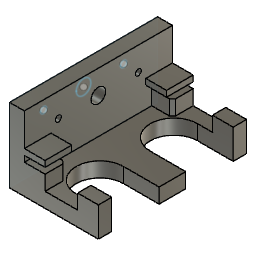
Ultrasonic sensor mount v1 (Autodesk Fusion 360 design; units mm, degrees)
Autodesk Fusion 360 part; units mm, degrees
sketch "Sketch1" plane through (0, 0, 0) normal (0, 0, 1) x (1, 0, 0)
  line L0 (0, 0) -> (30, 0)
  line L1 (30, 0) -> (30, 50)
  line L2 (30, 50) -> (0, 50)
  line L3 (0, 50) -> (0, 0)
  dimension "d1" = 30
  dimension "d2" = 50
  constraint horizontal L0
  constraint vertical L1
  constraint horizontal L2
  constraint vertical L3
  constraint coincident L0.start L3.end
  measures "d1" distance of L0.start L0.end
  measures "d2" distance of L0.start L2.end
extrude "Extrude1" add sketch "Sketch1" along normal blind 5
sketch "Sketch2" plane through (0, 0, 5) normal (0, 0, 1) x (-1, 0, 0)
  line L0 (0, -50) -> (0, 0)
  line L1 (0, 0) -> (-30, 0)
  line L2 (-30, 0) -> (-30, -50)
  line L3 (-30, -50) -> (0, -50)
  line L4 (0, -50) -> (-5, -50)
  line L5 (-5, -50) -> (-5, 0)
  line L6 (-5, 0) -> (0, 0)
  line L7 (0, 0) -> (0, -50)
  constraint horizontal L4
  constraint vertical L5
  constraint horizontal L6
  constraint vertical L7
  constraint coincident L0.start L3.end
extrude "Extrude2" add sketch "Sketch2" along normal blind 20 contours L0 L1 L3 L4 L5 L6 L7
sketch "Sketch3" plane through (0, 0, 5) normal (0, 0, 1) x (-1, 0, 0)
  line L0 (-5, -50) -> (-5, 0)
  line L1 (-5, 0) -> (-30, 0)
  line L2 (-30, 0) -> (-30, -50)
  line L3 (-30, -50) -> (-5, -50)
  line L4 (-30, 0) -> (-23, 0)
  line L5 (-23, 0) -> (-23, -7)
  line L6 (-23, -7) -> (-30, -7)
  line L7 (-30, -7) -> (-30, 0)
  line L8 (-30, -50) -> (-23, -50)
  line L9 (-23, -50) -> (-23, -43)
  line L10 (-23, -43) -> (-30, -43)
  line L11 (-30, -43) -> (-30, -50)
  line L12 (-5, -50) -> (-12, -50)
  line L13 (-12, -50) -> (-12, -43)
  line L14 (-12, -43) -> (-5, -43)
  line L15 (-5, -43) -> (-5, -50)
  line L16 (-5, 0) -> (-12, 0)
  line L17 (-12, 0) -> (-12, -7)
  line L18 (-12, -7) -> (-5, -7)
  line L19 (-5, -7) -> (-5, 0)
  circle A0 centre (-18, -12.5) radius 8
  circle A1 centre (-18, -37.5) radius 8
  dimension "d7" = 7
  dimension "d8" = 7
  dimension "d9" = 7
  dimension "d10" = 7
  dimension "d11" = 7
  dimension "d12" = 7
  dimension "d13" = 7
  dimension "d14" = 7
  dimension "d16" = 16
  dimension "d17" = 16
  constraint horizontal L4
  constraint vertical L5
  constraint horizontal L6
  constraint vertical L7
  constraint coincident L1.end L2.start
  constraint horizontal L8
  constraint vertical L9
  constraint horizontal L10
  constraint vertical L11
  constraint coincident L2.end L3.start
  constraint horizontal L12
  constraint vertical L13
  constraint horizontal L14
  constraint vertical L15
  constraint coincident L0.start L3.end
  constraint horizontal L16
  constraint vertical L17
  constraint horizontal L18
  constraint vertical L19
  constraint coincident L0.end L1.start
  measures "d7" distance of L1.end L4.end
  measures "d8" distance of L1.end L6.end
  measures "d9" distance of L2.end L8.end
  measures "d10" distance of L2.end L10.end
  measures "d11" distance of L0.start L12.end
  measures "d12" distance of L0.start L14.end
  measures "d13" distance of L0.end L16.end
  measures "d14" distance of L0.end L18.end
  measures "d16" diameter of A0
  measures "d17" diameter of A1
extrude "Extrude3" cut sketch "Sketch3" against normal blind 5 contours L9 L10 A1 | L5 L6 A0 picked at (-16.0576, -35.427) picked at (-16.0576, -14.573)
extrude "Extrude4" add sketch "Sketch3" along normal blind 5 contours L0 L3 L12 L13 L14 L15 | L0 L1 L16 L17 L18 L19 | L2 L3 L8 L9 L10 L11 A1 | L1 L2 L4 L5 L6 L7 A0
extrude "Extrude5" cut sketch "Sketch3" against normal blind 5 contours L9 L10 A1 | L5 L6 A0 picked at (-23.2774, -43.2566) picked at (-23.2774, -6.7434)
chamfer "Chamfer1" distance 1 angle 45 2 edges at (12, 7, 7.5) (12, 43, 7.5)
sketch "Sketch4" plane through (30, 0, 0) normal (1, 0, 0) x (0, 1, 0)
  line L0 (0, 0) -> (50, 0)
  line L1 (50, 0) -> (50, 10)
  line L2 (50, 10) -> (43, 10)
  line L3 (43, 10) -> (43, 5)
  line L4 (43, 5) -> (7, 5)
  line L5 (7, 5) -> (7, 10)
  line L6 (7, 10) -> (0, 10)
  line L7 (0, 10) -> (0, 0)
  line L8 (20.5, 5.0863) -> (4.5107, 5.0863)
  line L9 (4.5107, 5.0863) -> (4.5107, 0)
  line L10 (4.5107, 0) -> (20.5, 0)
  line L11 (20.5, 0) -> (20.5, 5.0863)
  line L12 (29.4867, 0) -> (45.5, 0)
  line L13 (45.5, 0) -> (45.5, 5.0968)
  line L14 (45.5, 5.0968) -> (29.4867, 5.0968)
  line L15 (29.4867, 5.0968) -> (29.4867, 0)
  line L16 (7, 10) -> (4.5107, 10)
  line L17 (4.5107, 10) -> (4.5107, 5.0863)
  line L18 (4.5107, 5.0863) -> (7, 5.0863)
  line L19 (7, 5.0863) -> (7, 10)
  line L20 (43, 10) -> (45.5, 10)
  line L21 (45.5, 10) -> (45.5, 5.0968)
  line L22 (45.5, 5.0968) -> (43, 5.0968)
  line L23 (43, 5.0968) -> (43, 10)
  constraint horizontal L8
  constraint vertical L9
  constraint horizontal L10
  constraint vertical L11
  constraint coincident L0 L9.end
  constraint horizontal L12
  constraint vertical L13
  constraint horizontal L14
  constraint vertical L15
  constraint coincident L0 L12.start
  constraint horizontal L16
  constraint vertical L17
  constraint horizontal L18
  constraint vertical L19
  constraint coincident L5.end L6.start
  constraint horizontal L20
  constraint vertical L21
  constraint horizontal L22
  constraint vertical L23
  constraint coincident L2.end L3.start
extrude "Extrude6" cut sketch "Sketch4" against normal blind 12 contours L0 L4 L5 L8 L9 L10 L11 L18 | L5 L6 L8 L16 L17 L18 L19 | L0 L3 L4 L12 L13 L14 L15 L22 | L2 L3 L14 L20 L21 L22 L23
sketch "Sketch5" plane through (0, 0, 0) normal (-1, 0, 0) x (0, -1, 0)
  line L0 (-50, 0) -> (0, 0)
  line L1 (0, 0) -> (0, 25)
  line L2 (0, 25) -> (-50, 25)
  line L3 (-50, 25) -> (-50, 0)
  circle A0 centre (-25, 17) radius 2.45
  circle A1 centre (-38.5, 17) radius 1
  circle A2 centre (-11.5, 17) radius 1
  dimension "d27" = 4.9
  dimension "d36" = 2
  dimension "d37" = 2
  measures "d27" diameter of A0
  measures "d36" diameter of A1
  measures "d37" diameter of A2
extrude "Extrude7" cut sketch "Sketch5" against normal blind 5 contours A0 | A1 | A2
sketch "Sketch6" plane through (5, 0, 0) normal (1, 0, 0) x (0, 1, 0)
  circle A0 centre (25, 17) radius 2.45
  line L0 (0, 10) -> (7, 10)
  line L1 (7, 10) -> (7, 5)
  line L2 (7, 5) -> (43, 5)
  line L3 (43, 5) -> (43, 10)
  line L4 (43, 10) -> (50, 10)
  line L5 (50, 10) -> (50, 25)
  line L6 (50, 25) -> (0, 25)
  line L7 (0, 25) -> (0, 10)
  line L8 (0, 12) -> (9, 12)
  line L9 (9, 12) -> (9, 14)
  line L10 (9, 14) -> (0, 14)
  line L11 (0, 14) -> (0, 12)
  line L12 (50, 12) -> (41, 12)
  line L13 (41, 12) -> (41, 14)
  line L14 (41, 14) -> (50, 14)
  line L15 (50, 14) -> (50, 12)
  circle A1 centre (11.5, 17) radius 1
  circle A2 centre (38.5, 17) radius 1
  constraint horizontal L8
  constraint vertical L9
  constraint horizontal L10
  constraint vertical L11
  constraint horizontal L12
  constraint vertical L13
  constraint horizontal L14
  constraint vertical L15
extrude "Extrude8" add sketch "Sketch6" along normal blind 7 contours L7 L8 L9 L10 L11 | L5 L12 L13 L14 L15
